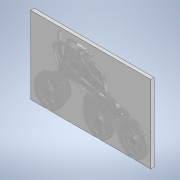
# Autodesk Inventor part: Rover 3 - Verde2
Saved by Autodesk Inventor 2020.1 (Build 241239000, 239)
## iProperties
Created: 2020-06-20
Part Number: Rover 3 - Verde2
Material: Genérico
Document SubType Name: Modeling
Designer: rotje
Density: 1 g/cm^3
Appearance: Valor por defecto
Author: rotje
Autodesk Inventor part; units mm, degrees
ref_plane "YZ Plane" through (0, 0, 0) normal (1, 0, 0) x (0, 1, 0)
ref_plane "XZ Plane" through (0, 0, 0) normal (0, 1, 0) x (-1, 0, 0)
ref_plane "XY Plane" through (0, 0, 0) normal (0, 0, 1) x (1, 0, 0)
sketch "Boceto1" plane through (41.0474, 75.5331, 0) normal (0, 0, -1) x (-1, 0, 0)
  line L0 (50.1315, -75.5331) -> (-158.224, -75.5331)
  line L1 (-158.224, -75.5331) -> (-158.224, 58.9532)
  line L2 (-158.224, 58.9532) -> (50.1315, 58.9532)
  line L3 (50.1315, 58.9532) -> (50.1315, -75.5331)
  point P0 (41.0474, -75.5331)
  constraints: 8 end point, 2 parallel, 1 horizontal, 1 perpendicular
extrude "Extrusión1" add sketch "Boceto1" along normal blind 1.75 and the other way blind 4.25
